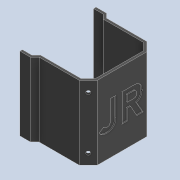
# Autodesk Inventor part: Z Axis Cover Top Logo
Saved by Autodesk Inventor 2022 (Build 260153000, 153)
## iProperties
Created: 2021-10-26
Part Number: Z Axis Cover Top Logo
Material: Generic
Document SubType Name: Modeling
Designer: Coy
Density: 1 g/cm^3
Appearance: Generic
Author: Coy
Autodesk Inventor part; units mm, degrees
ref_plane "YZ Plane" through (0, 0, 0) normal (1, 0, 0) x (0, 1, 0)
ref_plane "XZ Plane" through (0, 0, 0) normal (0, 1, 0) x (-1, 0, 0)
sketch "Sketch1" plane through (0, 0, 0) normal (0, 1, 0) x (-1, 0, 0)
  line L0 (0, 0) -> (0, 68.2)
  line L1 (0, 68.2) -> (10.6066, 78.8066)
  line L2 (10.6066, 78.8066) -> (68.3066, 78.8066)
  line L3 (68.3066, 78.8066) -> (74.5, 85)
  line L4 (74.5, 85) -> (88, 85)
  line L5 (0, 34.1) -> (80, 34.1) construction
  line L6 (0, 0) -> (10.6066, -10.6066)
  line L7 (10.6066, -10.6066) -> (68.3066, -10.6066)
  line L8 (68.3066, -10.6066) -> (74.5, -16.8)
  line L9 (74.5, -16.8) -> (88, -16.8)
  line L10 (88, 88.5) -> (73.0503, 88.5)
  line L11 (73.0503, 88.5) -> (66.8569, 82.3066)
  line L12 (66.8569, 82.3066) -> (9.1569, 82.3066)
  line L13 (9.1569, 82.3066) -> (-3.5, 69.6497)
  line L14 (-3.5, 69.6497) -> (-3.5, -1.4497)
  line L15 (-3.5, -1.4497) -> (9.1569, -14.1066)
  line L16 (9.1569, -14.1066) -> (66.8569, -14.1066)
  line L17 (66.8569, -14.1066) -> (73.0503, -20.3)
  line L18 (73.0503, -20.3) -> (88, -20.3)
  line L19 (88, 88.5) -> (88, 85)
  line L20 (88, -16.8) -> (88, -20.3)
  dimension "d0" = 68.2
  dimension "d1" = 15
  dimension "d2" = 135
  dimension "d5" = 135
  dimension "d6" = 88
  dimension "d7" = 3.5
  dimension "d18" = 13.5
  dimension "d19" = 50.9
  constraints: 42 end point, 4 parallel, 4 symmetric about line, 2 perpendicular, 2 vertical, 1 collinear, 1 horizontal, 1 midpoint, 8 other
  measures "d0" distance of L0.start L0.end
  measures "d1" distance of L0.end L1.end
  measures "d2" angle of L0 L1
  measures "d5" angle of L3 L2
  measures "d6" horizontal distance of L0.start L4.end
  measures "d7" distance between parallel lines of L3 L11
  measures "d18" distance of L3.end L4.end
  measures "d19" distance between parallel lines of L5 L4
extrude "Extrusion1" add sketch "Sketch1" along normal blind 105
sketch "Sketch2" plane through (3.5, 0, 69.6497) normal (0.7071068, 0, 0.7071068) x (0.7071068, 0, -0.7071068)
  line L0 (-17.8995, 0) -> (0, 0) projected
  line L1 (0, 0) -> (0, 105) projected
  line L2 (-17.8995, 105) -> (0, 105) projected
  line L3 (-17.8995, 0) -> (-17.8995, 105) projected
  line L4 (-1.4497, 105) -> (-16.4497, 105) construction
  line L5 (-8.9497, 105) -> (-8.9497, 0) construction
  line L6 (-17.8995, 0) -> (0, 0) construction
  circle A0 centre (-8.9497, 90) radius 2.6
  circle A1 centre (-8.9497, 15) radius 2.6
  point P0 (46.7749, 0)
  dimension "d10" = 5.2
  dimension "d11" = 5.2
  dimension "d12" = 15
  dimension "d13" = 15
  constraints: 2 centre point, 2 end point, 2 midpoint, 2 point on line
  measures "d10" diameter of A0
  measures "d11" diameter of A1
  measures "d12" distance from line of L2 A0.centre
  measures "d13" distance from line of L0 A1.centre
extrude "Extrusion2" cut sketch "Sketch2" against normal up to next contours A0 | A1
ref_plane "Work Plane1" through (-88, 0, 34.1) normal (0, 0, 1) x (1, 0, 0)
mirror "Mirror1" about plane through (-88, 0, 34.1) normal (0, 0, 1) of "Extrusion2"
sketch "Sketch3" plane through (3.5, 0, 69.6497) normal (1, 0, 0) x (0, 0, -1)
  line L0 (0, 0) -> (71.0995, 0) construction
  line L1 (71.0995, 0) -> (71.0995, 105) construction
  line L2 (0, 105) -> (71.0995, 105) construction
  line L3 (0, 0) -> (0, 105) construction
  line L4 (0.5481, 104.9771) -> (70.0913, 104.9771) construction
  line L5 (70.0913, 104.9771) -> (70.0913, 0.7727) construction
  line L6 (70.0913, 0.7727) -> (0.5481, 0.7727) construction
  line L7 (0.5481, 0.7727) -> (0.5481, 104.9771) construction
  spline S0 degree 2 poles (14.015, 32.6767) (10.3486, 32.6767) (4.6013, 35.5174) (2.9828, 38.1268) knots 0 0 0 1 2 2 2
  line L8 (2.9828, 38.1268) -> (9.1595, 42.6189)
  spline S1 degree 2 poles (9.1595, 42.6189) (10.1504, 41.3638) (12.925, 39.9765) (14.4444, 39.9765) knots 0 0 0 1 2 2 2
  spline S2 degree 2 poles (14.4444, 39.9765) (16.6244, 39.9765) (18.9696, 43.0483) (18.9696, 45.8229) knots 0 0 0 1 2 2 2
  line L9 (18.9696, 45.8229) -> (18.9696, 73.0731)
  line L10 (18.9696, 73.0731) -> (26.7978, 73.0731)
  line L11 (26.7978, 73.0731) -> (26.7978, 45.7899)
  spline S3 degree 2 poles (26.7978, 45.7899) (26.7978, 41.628) (23.792, 35.7486) (18.0777, 32.6767) (14.015, 32.6767) knots 0 0 0 1 2 3 3 3
  line L12 (38.5897, 56.4257) -> (52.5286, 56.4257)
  spline S4 degree 2 poles (52.5286, 56.4257) (53.6847, 56.4257) (55.4353, 57.5818) (56.3932, 59.7287) (56.4262, 61.1491) knots 0 0 0 1 2 3 3 3
  spline S5 degree 2 poles (56.4262, 61.1491) (56.4262, 62.5363) (55.4683, 64.6833) (53.6847, 65.8394) (52.5286, 65.8394) knots 0 0 0 1 2 3 3 3
  line L13 (52.5286, 65.8394) -> (38.5897, 65.8394)
  line L14 (38.5897, 65.8394) -> (38.5897, 73.1061)
  line L15 (38.5897, 73.1061) -> (53.1232, 73.1061)
  spline S6 degree 2 poles (53.1232, 73.1061) (56.4262, 73.1061) (61.4138, 70.1334) (64.1884, 64.7164) (64.1884, 61.1491) knots 0 0 0 1 2 3 3 3
  spline S7 degree 2 poles (64.1884, 61.1491) (64.1884, 57.5487) (61.4138, 52.1317) (56.3932, 49.159) (53.1232, 49.159) knots 0 0 0 1 2 3 3 3
  line L16 (53.1232, 49.159) -> (38.5897, 49.159)
  line L17 (38.5897, 49.159) -> (38.5897, 56.4257)
  line L18 (35.5839, 73.1061) -> (43.1479, 73.1061)
  line L19 (43.1479, 73.1061) -> (43.1479, 33.0731)
  line L20 (43.1479, 33.0731) -> (35.5839, 33.0731)
  line L21 (35.5839, 33.0731) -> (35.5839, 73.1061)
  line L22 (47.0125, 50.4141) -> (55.072, 51.6693)
  line L23 (55.072, 51.6693) -> (65.873, 33.0731)
  line L24 (65.873, 33.0731) -> (56.7235, 33.0731)
  line L25 (56.7235, 33.0731) -> (47.0125, 50.4141)
  point P0 (69.6497, 0)
  constraints: 2 other
extrude "Extrusion3" cut sketch "Sketch3" against normal blind 1.5 contours S0 L8 S1 S2 L9 L10 L11 S3 | L17 L16 L19 L20 L21 L18 L14 L13 L12 | L12 L19 L16 L17 | L12 S4 S5 L13 L19 L15 S6 S7 L23 L22 L25 L16 | L13 L14 L15 L19 | L25 L22 L23 S7 L16 | L16 S7 L23 L24 L25
sketch "Sketch4" plane through (-10.6066, 0, 78.8066) normal (0, 0, -1) x (-1, 0, 0)
  line L0 (27.7, 12) -> (42.7, 12)
  line L1 (42.7, 12) -> (42.7, 0)
  line L2 (42.7, 0) -> (27.7, 0)
  line L3 (27.7, 0) -> (27.7, 12)
  line L4 (0, 0) -> (57.7, 0) projected
  line L5 (57.7, 0) -> (57.7, 105) projected
  point P0 (-10.6066, 0)
  dimension "d20" = 15
  dimension "d21" = 12
  dimension "d22" = 15
  constraints: 8 end point, 2 parallel, 1 collinear, 1 horizontal, 1 perpendicular
  measures "d20" distance of L1.end L2.end
  measures "d21" distance of L0.end L1.end
  measures "d22" distance between parallel lines of L5 L1
extrude "Extrusion4" add sketch "Sketch4" along normal blind 6
sketch "Sketch5" plane through (-53.3066, 0, 78.8066) normal (-1, 0, 0) x (0, 0, 1)
  line L0 (0, 12) -> (0, 0) projected
  line L1 (0, 12) -> (-6, 12) projected
  line L2 (-6, 0) -> (-6, 12) projected
  line L3 (0, 0) -> (-6, 0) projected
  line L4 (-3.75, 7) -> (-2.25, 7)
  line L5 (-2.25, 7) -> (-2.25, 5)
  line L6 (-2.25, 5) -> (-3.75, 5)
  line L7 (-3.75, 5) -> (-3.75, 7)
  line L8 (0, 12) -> (-6, 12) construction
  line L9 (-3, 12) -> (-3, 7) construction
  line L10 (-3.75, 6) -> (-6, 6) construction
  line L11 (-6, 12) -> (-6, 0) construction
  line L12 (0, 12) -> (-6, 12) construction
  line L13 (-6, 0) -> (-6, 12) construction
  point P0 (-78.8066, 0)
  dimension "d25" = 1.5
  dimension "d26" = 2
  constraints: 12 end point, 4 midpoint, 3 perpendicular, 2 parallel, 1 horizontal
  measures "d25" distance of L5.end L6.end
  measures "d26" distance of L4.end L5.end
extrude "Extrusion5" cut sketch "Sketch5" against normal up to next contours L4 L5 L6 L7
chamfer "Chamfer1" distance 3 distance2 6 1 edges at (-53.3066, 6, 72.8066)
chamfer "Chamfer2" distance 3 distance2 6 1 edges at (-38.3066, 6, 72.8066)
fillet "Fillet1" radius 6 2 edges at (-45.8066, 12, 72.8066) (-45.8066, 0, 72.8066)
equation "\"d11\" = d10"
equation "\"d13\" = d12"
body "Solid1"
